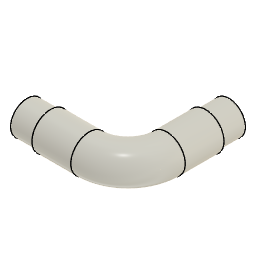
90° Rod Connector (Autodesk Fusion 360 design; units mm, degrees)
Autodesk Fusion 360 part; units mm, degrees
sketch "Sketch1" plane through (0, 0, 0) normal (0, 0, 1) x (1, 0, 0)
  line L0 (0, 0) -> (50, 0)
  line L1 (75, 25) -> (75, 75)
  arc A0 (50, 0) -> (75, 25) centre (50, 25) ccw
  point P0 (75, 0)
  dimension "d1" = 75
  dimension "d2" = 75
  dimension "d3" = 25
  constraint coincident L0.start origin
  constraint horizontal L0
  constraint perpendicular L0 L1
  constraint coincident P0 L0
  constraint coincident P0 L1
  constraint tangent L0 A0
  constraint tangent L1 A0
  measures "d1" distance of L0.start P0
  measures "d2" distance of P0 L1.end
  measures "d3" radius of A0
pipe "Pipe1" add diameter 23.75 path "Sketch1" along L1 A0 L0 makes body 1
move_face "OffsetFaces1" offset -25 1 faces at (78.5573, 75, 3.7042) on bodies 1
move_face "OffsetFaces2" offset -25 1 faces at (0, -3.5573, 3.7042) on bodies 1
cylinder "CylinderPrimitive1" add diameter 21.25 height 15 placed x (1, 0, 0) y (0, 0, -1) z (0, 1, 0) at (75, 50, 0) separate body makes body 2
cylinder "CylinderPrimitive2" add diameter 21.25 height 15 placed x (0, 0, 1) y (0, 1, 0) z (-1, 0, 0) at (25, 0, 0) separate body makes body 3
